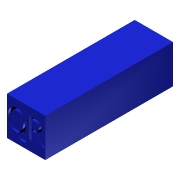
# Autodesk Inventor part: Container 1 1 5
Saved by Autodesk Inventor 2015 (Build 190159000, 159)
## iProperties
Created: 2015-03-07
Part Number: Container 1 1 5
Material: Generic
Document SubType Name: Modeling
Designer: Vukica
Density: 1 g/cm^3
Appearance: Blue - Wall Paint - Glossy
Author: Vukica
Autodesk Inventor part; units mm, degrees
ref_plane "YZ Plane" through (0, 0, 0) normal (1, 0, 0) x (0, 1, 0)
ref_plane "XZ Plane" through (0, 0, 0) normal (0, 1, 0) x (-1, 0, 0)
ref_plane "XY Plane" through (0, 0, 0) normal (0, 0, 1) x (1, 0, 0)
sketch "Sketch1" plane through (0, 0, 0) normal (0, 0, 1) x (1, 0, 0)
  line L0 (0, 0) -> (38.1, 0)
  line L1 (38.1, 0) -> (38.1, 38.1)
  line L2 (38.1, 38.1) -> (0, 38.1)
  line L3 (0, 38.1) -> (0, 0)
  dimension "d0" = 38.1
  dimension "d1" = 38.1
  constraints: 8 end point, 2 parallel, 1 horizontal, 1 perpendicular
  measures "d0" distance of L1.end L2.end
  measures "d1" distance of L2.end L0.start
extrude "Extrusion1" add sketch "Sketch1" along normal blind 127
sketch "Sketch2" plane through (0, 0, 127) normal (0, 0, 1) x (1, 0, 0)
  line L0 (0.0378, 30.7796) -> (46.433, 30.7796) construction
  line L1 (46.433, 30.7796) -> (46.433, -1.8452) construction
  line L2 (46.433, -1.8452) -> (0.0378, -1.8452) construction
  line L3 (0.0378, -1.8452) -> (0.0378, 30.7796) construction
  spline S0 degree 2 poles (18.9746, 5.0585) (18.2336, 4.8773) (16.6199, 4.6797) (15.813, 4.6797) knots 0 0 0 1 2 2 2
  spline S1 degree 2 poles (15.813, 4.6797) (13.5241, 4.6797) (10.6754, 7.2321) (10.5436, 9.6033) knots 0 0 0 1 2 2 2
  spline S2 degree 2 poles (10.5436, 9.6033) (10.3625, 9.6033) (10.0496, 9.6033) (9.9179, 9.6033) knots 0 0 0 1 2 2 2
  spline S3 degree 2 poles (9.9179, 9.6033) (7.8595, 9.6033) (4.5497, 11.003) (3.3641, 12.3697) knots 0 0 0 1 2 2 2
  spline S4 degree 2 poles (3.3641, 12.3697) (2.195, 13.72) (0.9435, 17.672) (0.9435, 20.175) knots 0 0 0 1 2 2 2
  spline S5 degree 2 poles (0.9435, 20.175) (0.9435, 22.7438) (2.2114, 26.6299) (3.3806, 28.0131) knots 0 0 0 1 2 2 2
  spline S6 degree 2 poles (3.3806, 28.0131) (4.5662, 29.3799) (7.876, 30.7796) (9.9179, 30.7796) knots 0 0 0 1 2 2 2
  spline S7 degree 2 poles (9.9179, 30.7796) (11.9927, 30.7796) (15.319, 29.3305) (16.4717, 28.0131) knots 0 0 0 1 2 2 2
  spline S8 degree 2 poles (16.4717, 28.0131) (17.6243, 26.6793) (18.9087, 22.7108) (18.9087, 20.175) knots 0 0 0 1 2 2 2
  spline S9 degree 2 poles (18.9087, 20.175) (18.9087, 16.2229) (15.8295, 11.0853) (13.1454, 10.1796) knots 0 0 0 1 2 2 2
  spline S10 degree 2 poles (13.1454, 10.1796) (13.2112, 9.4222) (13.6064, 8.2036) (13.9193, 7.8578) knots 0 0 0 1 2 2 2
  spline S11 degree 2 poles (13.9193, 7.8578) (14.298, 7.4297) (15.3355, 7.0345) (16.2576, 7.0345) knots 0 0 0 1 2 2 2
  spline S12 degree 2 poles (16.2576, 7.0345) (16.801, 7.0345) (18.283, 7.3803) (18.6123, 7.512) knots 0 0 0 1 2 2 2
  line L4 (18.6123, 7.512) -> (18.9746, 7.512)
  line L5 (18.9746, 7.512) -> (18.9746, 5.0585)
  spline S13 degree 2 poles (16.0929, 20.175) (16.0929, 22.2004) (15.2202, 25.3126) (14.4298, 26.3335) knots 0 0 0 1 2 2 2
  spline S14 degree 2 poles (14.4298, 26.3335) (13.6229, 27.3874) (11.3505, 28.4413) (9.9343, 28.4413) knots 0 0 0 1 2 2 2
  spline S15 degree 2 poles (9.9343, 28.4413) (8.4688, 28.4413) (6.2623, 27.4203) (5.4225, 26.3335) knots 0 0 0 1 2 2 2
  spline S16 degree 2 poles (5.4225, 26.3335) (4.6156, 25.2961) (3.7593, 22.151) (3.7593, 20.175) knots 0 0 0 1 2 2 2
  spline S17 degree 2 poles (3.7593, 20.175) (3.7593, 16.1735) (7.1185, 11.9086) (9.9343, 11.9086) knots 0 0 0 1 2 2 2
  spline S18 degree 2 poles (9.9343, 11.9086) (12.7502, 11.9086) (16.0929, 16.1735) (16.0929, 20.175) knots 0 0 0 1 2 2 2
  line L6 (37.5985, 10.0314) -> (34.0911, 10.0314)
  line L7 (34.0911, 10.0314) -> (27.6691, 18.1166)
  line L8 (27.6691, 18.1166) -> (24.5733, 18.1166)
  line L9 (24.5733, 18.1166) -> (24.5733, 10.0314)
  line L10 (24.5733, 10.0314) -> (21.8728, 10.0314)
  line L11 (21.8728, 10.0314) -> (21.8728, 30.3514)
  line L12 (21.8728, 30.3514) -> (27.1092, 30.3514)
  spline S19 degree 2 poles (27.1092, 30.3514) (28.8547, 30.3514) (31.2094, 29.9727) (32.2798, 29.2811) knots 0 0 0 1 2 2 2
  spline S20 degree 2 poles (32.2798, 29.2811) (33.3501, 28.5895) (34.5851, 26.4323) (34.5851, 24.8351) knots 0 0 0 1 2 2 2
  spline S21 degree 2 poles (34.5851, 24.8351) (34.5851, 22.612) (32.3127, 19.5986) (30.3696, 18.8741) knots 0 0 0 1 2 2 2
  line L13 (30.3696, 18.8741) -> (37.5985, 10.0314)
  spline S22 degree 2 poles (31.7693, 24.621) (31.7693, 25.5102) (31.1436, 26.8769) (30.4849, 27.3215) knots 0 0 0 1 2 2 2
  spline S23 degree 2 poles (30.4849, 27.3215) (29.9085, 27.7003) (28.3771, 28.0131) (27.2574, 28.0131) knots 0 0 0 1 2 2 2
  line L14 (27.2574, 28.0131) -> (24.5733, 28.0131)
  line L15 (24.5733, 28.0131) -> (24.5733, 20.3726)
  line L16 (24.5733, 20.3726) -> (26.9445, 20.3726)
  spline S24 degree 2 poles (26.9445, 20.3726) (28.1137, 20.3726) (29.9744, 20.7842) (30.6166, 21.4264) knots 0 0 0 1 2 2 2
  spline S25 degree 2 poles (30.6166, 21.4264) (31.2094, 21.9863) (31.7693, 23.5671) (31.7693, 24.621) knots 0 0 0 1 2 2 2
  point P0 (0, 0)
  constraints: 2 other
extrude "Extrusion2" cut sketch "Sketch2" against normal blind 2.54
body "Solid1"
